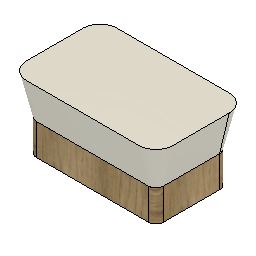
ZoomMuter_case_v13 (Autodesk Fusion 360 design; units mm, degrees)
Autodesk Fusion 360 part; units mm, degrees
note: some values were not read from the file. Set by a fixed rule: which sketch regions a step uses.
sketch "Sketch1" plane through (0, 0, 0) normal (0, 1, 0) x (1, 0, 0) in component "Case Front"
  line L0 (-27, 12.5) -> (-2, 12.5) construction
  line L1 (-2, 12.5) -> (-2, -12.5) construction
  line L2 (-2, -12.5) -> (-27, -12.5) construction
  line L3 (-27, -12.5) -> (-27, 12.5) construction
  line L4 (69.0491, 0) -> (-60.982, 0) construction
  line L5 (0, 36.3934) -> (0, -35.5501) construction
  line L6 (0, 18.5) -> (-33, 18.5)
  line L7 (-33, 18.5) -> (-33, 0)
  line L8 (-33, -18.5) -> (-33, 0)
  line L9 (0, -18.5) -> (-33, -18.5)
  line L10 (0, 18.5) -> (33, 18.5)
  line L11 (33, 18.5) -> (33, 0)
  line L12 (33, -18.5) -> (33, 0)
  line L13 (0, -18.5) -> (33, -18.5)
  line L14 (-14.5, 12.5) -> (-14.5, -12.5) construction
  line L15 (-7.2, -7.3) -> (-21.8, -7.3) construction
  line L16 (-21.8, -7.3) -> (-21.8, 7.3) construction
  line L17 (-21.8, 7.3) -> (-7.2, 7.3) construction
  line L18 (-7.2, 7.3) -> (-7.2, -7.3) construction
  line L19 (-7.2, -7.3) -> (-21.8, 7.3) construction
  line L20 (-21.8, -7.3) -> (-7.2, 7.3) construction
  line L21 (-22.1, 7.6) -> (-6.9, 7.6)
  line L22 (-6.9, 7.6) -> (-6.9, -7.6)
  line L23 (-6.9, -7.6) -> (-22.1, -7.6)
  line L24 (-22.1, -7.6) -> (-22.1, 7.6)
  line L25 (22.1, 7.6) -> (6.9, 7.6)
  line L26 (22.1, -7.6) -> (22.1, 7.6)
  line L27 (6.9, 7.6) -> (6.9, -7.6)
  line L28 (6.9, -7.6) -> (22.1, -7.6)
  line L29 (-22.7, 8.2) -> (-6.3, 8.2)
  line L30 (-6.3, 8.2) -> (-6.3, -8.2)
  line L31 (-6.3, -8.2) -> (-22.7, -8.2)
  line L32 (-22.7, -8.2) -> (-22.7, 8.2)
  line L33 (6.3, -8.2) -> (22.7, -8.2)
  line L34 (6.3, 8.2) -> (6.3, -8.2)
  line L35 (22.7, 8.2) -> (6.3, 8.2)
  line L36 (22.7, -8.2) -> (22.7, 8.2)
  point P0 (-14.5, 0)
  dimension "d1" = 25
  dimension "d2" = 25
  dimension "d5" = 6
  dimension "d6" = 6
  dimension "d7" = 6
  dimension "d11" = 14.6
  dimension "d12" = 14.6
  dimension "d14" = 2
  dimension "d39" = -0.9
  constraint horizontal L0
  constraint vertical L1
  constraint horizontal L2
  constraint vertical L3
  constraint perpendicular L1 L4
  constraint coincident origin L4
  constraint perpendicular L4 L5
  constraint coincident origin L5
  constraint coincident L5 L6.start
  constraint perpendicular L5 L6
  constraint coincident L4 L7.end
  constraint perpendicular L4 L7
  constraint symmetric L4 L6.start L9.start
  constraint symmetric L4 L6.end L8.start
  constraint symmetric L4 L7.end L8.end
  constraint symmetric L5 L6.start L10.start
  constraint symmetric L5 L6.end L10.end
  constraint symmetric L5 L7.end L11.end
  constraint symmetric L5 L8.start L12.start
  constraint symmetric L5 L9.start L13.start
  constraint midpoint L0 L14.start
  constraint midpoint L2 L14.end
  constraint perpendicular L15 L16
  constraint parallel L15 L17
  constraint parallel L16 L18
  constraint horizontal L15
  constraint coincident L19 P0
  constraint coincident L20 P0
  constraint midpoint L14 P0
  constraint symmetric L5 L21.start L25.start
  constraint symmetric L5 L21.end L25.end
  constraint symmetric L5 L22.end L27.end
  constraint symmetric L5 L23.end L26.start
  constraint symmetric L5 L29.start L35.start
  constraint symmetric L5 L29.end L34.start
  constraint symmetric L5 L30.end L33.start
  constraint symmetric L5 L31.end L33.end
  measures "d1" distance of L0.start L0.end
  measures "d2" distance of L0.start L2.end
  measures "d5" distance of L3 L7
  measures "d6" distance of L0 L6
  measures "d7" distance of L2 L9
  measures "d11" distance of L16.end L17.end
  measures "d12" distance of L15.end L16.end
  measures "d14" distance of L1 L5
extrude "Extrude1" add sketch "Sketch1" along normal blind 12 contours L6 L7 L8 L9 L10 L11 L12 L13 | L29 L30 L31 L32 | L33 L34 L35 L36 makes body 1 in component "Case Front"
extrude "Extrude5" cut sketch "Sketch1" along normal blind 10.5 contours L29 L30 L31 L32 | L33 L34 L35 L36 bodies 1 in component "Case Front"
fillet "Fillet1" radius 4 4 edges at (-33, 6, -18.5) (-33, 6, 18.5) (33, 6, -18.5) (33, 6, 18.5) on bodies 1 in component "Case Front"
sketch "Sketch2" plane through (0, 12, 0) normal (0, 1, 0) x (-1, 0, 0) in component "Case Front"
  line L0 (-22.1, 7.6) -> (-6.9, 7.6)
  line L1 (-6.9, 7.6) -> (-6.9, -7.6)
  line L2 (-6.9, -7.6) -> (-22.1, -7.6)
  line L3 (-22.1, -7.6) -> (-22.1, 7.6)
  line L4 (6.9, 7.6) -> (22.1, 7.6)
  line L5 (22.1, 7.6) -> (22.1, -7.6)
  line L6 (22.1, -7.6) -> (6.9, -7.6)
  line L7 (6.9, -7.6) -> (6.9, 7.6)
  line L8 (29, 18.5) -> (-29, 18.5)
  line L9 (-33, 14.5) -> (-33, -14.5)
  line L10 (-29, -18.5) -> (29, -18.5)
  line L11 (33, -14.5) -> (33, 14.5)
  arc A0 (-29, 18.5) -> (-33, 14.5) centre (-29, 14.5) ccw
  arc A1 (-33, -14.5) -> (-29, -18.5) centre (-29, -14.5) ccw
  arc A2 (29, -18.5) -> (33, -14.5) centre (29, -14.5) ccw
  arc A3 (33, 14.5) -> (29, 18.5) centre (29, 14.5) ccw
  line L12 (31, -13.325) -> (31, 13.325)
  line L13 (27.825, 16.5) -> (-27.825, 16.5)
  line L14 (-31, 13.325) -> (-31, -13.325)
  line L15 (-27.825, -16.5) -> (27.825, -16.5)
  arc A4 (27.825, -16.5) -> (31, -13.325) centre (27.825, -13.325) ccw
  arc A5 (-31, -13.325) -> (-27.825, -16.5) centre (-27.825, -13.325) ccw
  arc A6 (-27.825, 16.5) -> (-31, 13.325) centre (-27.825, 13.325) ccw
  arc A7 (31, 13.325) -> (27.825, 16.5) centre (27.825, 13.325) ccw
  line L16 (31.2, -13.325) -> (31.2, 13.325)
  arc A8 (31.2, 13.325) -> (27.825, 16.7) centre (27.825, 13.325) ccw
  line L17 (27.825, 16.7) -> (-27.825, 16.7)
  arc A9 (-27.825, 16.7) -> (-31.2, 13.325) centre (-27.825, 13.325) ccw
  line L18 (-31.2, 13.325) -> (-31.2, -13.325)
  arc A10 (-31.2, -13.325) -> (-27.825, -16.7) centre (-27.825, -13.325) ccw
  line L19 (-27.825, -16.7) -> (27.825, -16.7)
  arc A11 (27.825, -16.7) -> (31.2, -13.325) centre (27.825, -13.325) ccw
  dimension "d26" = 2
  dimension "d27" = 2
  dimension "d28" = 2
  dimension "d29" = 3.175
  dimension "d56" = 2
  dimension "d57" = 0.2
  constraint parallel L11 L12
  constraint parallel L8 L13
  constraint parallel L9 L14
  constraint tangent L12 A4
  constraint tangent L15 A4
  constraint tangent L14 A5
  constraint tangent L15 A5
  constraint equal A4 A5
  constraint tangent L14 A6
  constraint tangent L13 A6
  constraint equal A4 A6
  constraint tangent L13 A7
  constraint tangent L12 A7
  constraint equal A4 A7
  measures "d26" distance of L9 L14
  measures "d27" distance of L8 L13
  measures "d28" distance of L11 L12
  measures "d29" radius of A4
  measures "d56" distance of L10 L15
extrude "Extrude4" add sketch "Sketch2" along normal blind 4.2 contours L8 L9 L10 L11 A0 A1 A2 A3 bodies 1 in component "Case Front"
ref_plane "WorkPlane1" through (0, 12, 0) normal (0, 1, 0) x (0, 0, 1) in component "Switch Mockup"
sketch "Sketch1 (2)" plane through (0, 12, 0) normal (0, 1, 0) x (1, 0, 0) in component "Switch Mockup"
  line L0 (-6.9, -7.6) -> (-22.1, -7.6)
  line L1 (-22.1, -7.6) -> (-22.1, 7.6)
  line L2 (-6.9, 7.6) -> (-6.9, -7.6)
  line L3 (22.1, -7.6) -> (6.9, -7.6)
  line L4 (6.9, -7.6) -> (6.9, 7.6)
  line L5 (6.9, 7.6) -> (22.1, 7.6)
  line L6 (22.1, 7.6) -> (22.1, -7.6)
  line L7 (-6.9, -7.6) -> (-22.1, -7.6)
  line L8 (-22.1, -7.6) -> (-22.1, 7.6)
  line L9 (-22.1, 7.6) -> (-6.9, 7.6)
  line L10 (-6.9, 7.6) -> (-6.9, -7.6)
  line L11 (-31.2, 13.325) -> (-31.2, -13.325)
  arc A0 (-31.2, -13.325) -> (-27.825, -16.7) centre (-27.825, -13.325) ccw
  line L12 (-27.825, -16.7) -> (27.825, -16.7)
  arc A1 (27.825, -16.7) -> (31.2, -13.325) centre (27.825, -13.325) ccw
  line L13 (31.2, -13.325) -> (31.2, 13.325)
  arc A2 (31.2, 13.325) -> (27.825, 16.7) centre (27.825, 13.325) ccw
  line L14 (27.825, 16.7) -> (-27.825, 16.7)
  arc A3 (-27.825, 16.7) -> (-31.2, 13.325) centre (-27.825, 13.325) ccw
extrude "Extrude1'" add sketch "Sketch1 (2)" along normal blind 7.93 separate body contours L0 L1 L2 L7 L8 L9 L10 | L3 L4 L5 L6 makes body 2 at (-17.0333, 12, 2.5333) makes body 3 at (17.0333, 12, 2.5333) in component "Switch Mockup"
sketch "Sketch2 (2)" plane through (0, 19.93, 0) normal (0, 1, 0) x (-1, 0, 0) in component "Switch Mockup"
  line L0 (-22.1, -7.6) -> (-6.9, -7.6)
  line L1 (-6.9, -7.6) -> (-6.9, 7.6)
  line L2 (-6.9, 7.6) -> (-22.1, 7.6)
  line L3 (-22.1, 7.6) -> (-22.1, -7.6)
  circle A0 centre (15.2785, -5.9827) radius 1.0884
  circle A1 centre (15.2785, 4.052) radius 1.6496
  circle A2 centre (-14.7915, -5.9827) radius 0.7885
  circle A3 centre (-14.7915, 4.5657) radius 0.8169
extrude "Extrude2" add sketch "Sketch2 (2)" along normal blind 3.4 contours A0 | A1 | A2 | A3 bodies 2 3 in component "Switch Mockup"
ref_plane "WorkPlane1" through (0, 37, 0) normal (0, -1, 0) x (-1, 0, 0) in component "Case Back"
sketch "Sketch5" plane through (0, 16.2, 0) normal (0, 1, 0) x (-1, 0, 0) in component "Case Back"
  arc A0 (33, 14.5) -> (29, 18.5) centre (29, 14.5) ccw
  line L0 (29, 18.5) -> (-29, 18.5)
  arc A1 (-29, 18.5) -> (-33, 14.5) centre (-29, 14.5) ccw
  line L1 (-33, 14.5) -> (-33, -14.5)
  arc A2 (-33, -14.5) -> (-29, -18.5) centre (-29, -14.5) ccw
  line L2 (-29, -18.5) -> (29, -18.5)
  arc A3 (29, -18.5) -> (33, -14.5) centre (29, -14.5) ccw
  line L3 (33, -14.5) -> (33, 14.5)
  line L4 (-29, -18.5) -> (29, -18.5)
  arc A4 (29, -18.5) -> (33, -14.5) centre (29, -14.5) ccw
  line L5 (33, -14.5) -> (33, 14.5)
  arc A5 (33, 14.5) -> (29, 18.5) centre (29, 14.5) ccw
  line L6 (29, 18.5) -> (-29, 18.5)
  arc A6 (-29, 18.5) -> (-33, 14.5) centre (-29, 14.5) ccw
  line L7 (-33, 14.5) -> (-33, -14.5)
  arc A7 (-33, -14.5) -> (-29, -18.5) centre (-29, -14.5) ccw
sketch "Sketch4" plane through (0, 37, 0) normal (0, -1, 0) x (1, 0, 0) in component "Case Back"
  arc A0 (-29, 18.5) -> (-33, 14.5) centre (-29, 14.5) ccw
  line L0 (-29, 18.5) -> (29, 18.5)
  arc A1 (33, 14.5) -> (29, 18.5) centre (29, 14.5) ccw
  line L1 (33, 14.5) -> (33, -14.5)
  arc A2 (29, -18.5) -> (33, -14.5) centre (29, -14.5) ccw
  line L2 (29, -18.5) -> (-29, -18.5)
  arc A3 (-33, -14.5) -> (-29, -18.5) centre (-29, -14.5) ccw
  line L3 (-33, -14.5) -> (-33, 14.5)
  line L4 (29, -23.5) -> (-29, -23.5)
  arc A4 (-38, -14.5) -> (-29, -23.5) centre (-29, -14.5) ccw
  line L5 (-38, -14.5) -> (-38, 14.5)
  arc A5 (-29, 23.5) -> (-38, 14.5) centre (-29, 14.5) ccw
  line L6 (-29, 23.5) -> (29, 23.5)
  arc A6 (38, 14.5) -> (29, 23.5) centre (29, 14.5) ccw
  line L7 (38, 14.5) -> (38, -14.5)
  arc A7 (29, -23.5) -> (38, -14.5) centre (29, -14.5) ccw
  arc A8 (-29, 19.8) -> (-34.3, 14.5) centre (-29, 14.5) ccw
  line L8 (-34.3, -14.5) -> (-34.3, 14.5)
  arc A9 (-34.3, -14.5) -> (-29, -19.8) centre (-29, -14.5) ccw
  line L9 (29, -19.8) -> (-29, -19.8)
  arc A10 (29, -19.8) -> (34.3, -14.5) centre (29, -14.5) ccw
  line L10 (34.3, 14.5) -> (34.3, -14.5)
  arc A11 (34.3, 14.5) -> (29, 19.8) centre (29, 14.5) ccw
  line L11 (-29, 19.8) -> (29, 19.8)
  arc A12 (-31.2, -13.325) -> (-27.825, -16.7) centre (-27.825, -13.325) ccw
  line L12 (-27.825, -16.7) -> (27.825, -16.7)
  arc A13 (27.825, -16.7) -> (31.2, -13.325) centre (27.825, -13.325) ccw
  line L13 (31.2, -13.325) -> (31.2, 13.325)
  arc A14 (31.2, 13.325) -> (27.825, 16.7) centre (27.825, 13.325) ccw
  line L14 (27.825, 16.7) -> (-27.825, 16.7)
  arc A15 (-27.825, 16.7) -> (-31.2, 13.325) centre (-27.825, 13.325) ccw
  line L15 (-31.2, 13.325) -> (-31.2, -13.325)
  dimension "d33" = 5
  dimension "d35" = 1.3
loft "Loft1" add profiles "Sketch5", "Sketch4" section 1 section 2 contours L4 A4 L5 A5 L6 A6 L7 A7 separate body makes body 4 in component "Case Back"
shell "Shell2" thickness 3.7 removed faces 1 at (9.6667, 16.2, 6.1667) on bodies 4 in component "Case Back"
sketch "Sketch1 (3)" plane through (0, 16.2, 0) normal (0, 1, 0) x (-1, 0, 0) in component "Case Back"
  spline S0 degree 3 poles (-29.2013, -14.5) (-29.2013, -14.5015) (-29.2013, -14.506) (-29.2003, -14.5252) (-29.1983, -14.5383) (-29.1919, -14.5634) (-29.1875, -14.5752) (-29.1704, -14.6109) (-29.1539, -14.6321) (-29.1161, -14.6665) (-29.0934, -14.6807) (-29.0493, -14.6966) (-29.0305, -14.7) (-29.0089, -14.7011) (-29.0062, -14.7012) (-29.0025, -14.7013) (-29.0016, -14.7013) (-29.0005, -14.7013) (-29.0003, -14.7013) (-29, -14.7013) (-29, -14.7013) (-18.9136, -14.7013) (-9.2644, -14.7013) (5.7641, -14.7013) (11.2782, -14.7013) (19.004, -14.7013) (21.3301, -14.7013) (24.5877, -14.7013) (25.5676, -14.7013) (27.1216, -14.7013) (27.7083, -14.7013) (28.4749, -14.7013) (28.6696, -14.7013) (28.9056, -14.7013) (28.9526, -14.7013) (29.0022, -14.7013) (29.0085, -14.7012) (29.0298, -14.6997) (29.0426, -14.6974) (29.0674, -14.6905) (29.0791, -14.6859) (29.1146, -14.668) (29.1355, -14.6509) (29.1687, -14.6128) (29.1825, -14.5899) (29.1977, -14.5448) (29.2006, -14.5257) (29.2013, -14.5033) (29.2013, -14.5008) (29.2013, -9.4558) (29.2013, -4.6309) (29.2013, 2.8835) (29.2013, 5.6405) (29.2013, 9.5033) (29.2013, 10.6662) (29.2013, 12.4661) (29.2013, 13.1197) (29.2013, 14.0018) (29.2013, 14.2453) (29.2013, 14.4833) (29.2013, 14.4874) (29.2013, 14.5018) (29.2013, 14.5057) (29.2003, 14.5248) (29.1984, 14.5379) (29.192, 14.5631) (29.1877, 14.5748) (29.1707, 14.6105) (29.1542, 14.6318) (29.1164, 14.6663) (29.0937, 14.6805) (29.0497, 14.6965) (29.0309, 14.6999) (29.0094, 14.7011) (29.0066, 14.7012) (29.003, 14.7012) (29.002, 14.7013) (29.0005, 14.7013) (29, 14.7013) (13.9982, 14.7013) (-0.351, 14.7013) (-18.5064, 14.7013) (-22.6948, 14.7013) (-27.3011, 14.7013) (-27.8606, 14.7013) (-28.5398, 14.7013) (-28.6756, 14.7013) (-28.8435, 14.7013) (-28.8795, 14.7013) (-28.9316, 14.7013) (-28.9484, 14.7013) (-29.0028, 14.7013) (-29.005, 14.7013) (-29.0235, 14.7005) (-29.0366, 14.6986) (-29.0619, 14.6924) (-29.0737, 14.6881) (-29.1095, 14.6713) (-29.1308, 14.655) (-29.1656, 14.6174) (-29.1799, 14.5947) (-29.1962, 14.5509) (-29.1997, 14.5322) (-29.2013, 14.5066) (-29.2013, 14.4995) (-29.2013, 9.6328) (-29.2013, 4.8164) (-29.2013, 0) (-29.2013, -5.0431) (-29.2013, -9.8677) (-29.2013, -14.5) knots 1.51292242 1.51292242 1.51292242 1.51292242 1.51341061 1.51341061 1.51468048 1.51468048 1.51598415 1.51598415 1.51896361 1.51896361 1.52201263 1.52201263 1.52434216 1.52434216 1.52469932 1.52469932 1.52483423 1.52483423 1.52486538 1.52486538 1.52487073 1.52487073 1.86604744 1.86604744 2.07830234 2.07830234 2.17578069 2.17578069 2.2204858 2.2204858 2.2496217 2.2496217 2.26014609 2.26014609 2.26291297 2.26291297 2.26318968 2.26318968 2.26368981 2.26368981 2.26421181 2.26421181 2.26540782 2.26540782 2.26659472 2.26659472 2.26750254 2.26750254 2.26767067 2.26767067 2.77651558 2.77651558 3.09305783 3.09305783 3.23842388 3.23842388 3.32736932 3.32736932 3.36344051 3.36344051 3.36409413 3.36409413 3.36586679 3.36586679 3.37067589 3.37067589 3.37560507 3.37560507 3.38686687 3.38686687 3.39841677 3.39841677 3.4072384 3.4072384 3.40858843 3.40858843 3.409115 3.409115 3.40942694 3.40942694 5.06474265 5.06474265 5.59075846 5.59075846 5.66725479 5.66725479 5.68746684 5.68746684 5.69329523 5.69329523 5.69626231 5.69626231 5.70328303 5.70328303 5.72519357 5.72519357 5.74753972 5.74753972 5.79854212 5.79854212 5.8511881 5.8511881 5.89135844 5.89135844 5.90648228 5.90648228 7.35139546 7.35139546 7.35139546 8.86431788 8.86431788 8.86431788 8.86431788
  spline S1 degree 3 poles (-33, -14.5) (-33, -15.0365) (-32.8906, -15.5727) (-32.6806, -16.0663) (-32.5243, -16.4335) (-32.3127, -16.7771) (-32.0551, -17.0819) (-31.6766, -17.5299) (-31.1981, -17.893) (-30.6648, -18.1371) (-30.1444, -18.3753) (-29.5724, -18.5) (-29, -18.5) (-16.7583, -18.5) (16.7583, -18.5) (29, -18.5) (29.5365, -18.5) (30.0727, -18.3906) (30.5663, -18.1806) (30.9335, -18.0243) (31.2771, -17.8127) (31.5819, -17.5551) (32.0299, -17.1766) (32.393, -16.6981) (32.6371, -16.1648) (32.8753, -15.6444) (33, -15.0724) (33, -14.5) (33, -8.3792) (33, 8.3792) (33, 14.5) (33, 15.0365) (32.8906, 15.5727) (32.6806, 16.0663) (32.5243, 16.4335) (32.3127, 16.7771) (32.0551, 17.0819) (31.6766, 17.5299) (31.1981, 17.893) (30.6648, 18.1371) (30.1444, 18.3753) (29.5724, 18.5) (29, 18.5) (16.7583, 18.5) (-16.7583, 18.5) (-29, 18.5) (-29.5365, 18.5) (-30.0727, 18.3906) (-30.5663, 18.1806) (-30.9335, 18.0243) (-31.2771, 17.8127) (-31.5819, 17.5551) (-32.0299, 17.1766) (-32.393, 16.6981) (-32.6371, 16.1648) (-32.8753, 15.6444) (-33, 15.0724) (-33, 14.5) (-33, 8.3792) (-33, -8.3792) (-33, -14.5) knots 0 0 0 0 0.011894 0.011894 0.011894 0.020742 0.020742 0.020742 0.033746 0.033746 0.033746 0.046436 0.046436 0.046436 0.317855 0.317855 0.317855 0.329749 0.329749 0.329749 0.338597 0.338597 0.338597 0.351601 0.351601 0.351601 0.364291 0.364291 0.364291 0.5 0.5 0.5 0.511894 0.511894 0.511894 0.520742 0.520742 0.520742 0.533746 0.533746 0.533746 0.546436 0.546436 0.546436 0.817855 0.817855 0.817855 0.829749 0.829749 0.829749 0.838597 0.838597 0.838597 0.851601 0.851601 0.851601 0.864291 0.864291 0.864291 1 1 1 1
  arc A0 (27.825, -16.5) -> (31, -13.325) centre (27.825, -13.325) ccw
  line L0 (-27.825, -16.5) -> (27.825, -16.5)
  line L1 (31, -13.325) -> (31, 13.325)
  arc A1 (31, 13.325) -> (27.825, 16.5) centre (27.825, 13.325) ccw
  line L2 (27.825, 16.5) -> (-27.825, 16.5)
  arc A2 (-27.825, 16.5) -> (-31, 13.325) centre (-27.825, 13.325) ccw
  line L3 (-31, 13.325) -> (-31, -13.325)
  arc A3 (-31, -13.325) -> (-27.825, -16.5) centre (-27.825, -13.325) ccw
  line L4 (30.8, -13.325) -> (30.8, 13.325)
  arc A4 (30.8, 13.325) -> (27.825, 16.3) centre (27.825, 13.325) ccw
  line L5 (27.825, 16.3) -> (-27.825, 16.3)
  arc A5 (-27.825, 16.3) -> (-30.8, 13.325) centre (-27.825, 13.325) ccw
  line L6 (-30.8, 13.325) -> (-30.8, -13.325)
  arc A6 (-30.8, -13.325) -> (-27.825, -16.3) centre (-27.825, -13.325) ccw
  line L7 (-27.825, -16.3) -> (27.825, -16.3)
  arc A7 (27.825, -16.3) -> (30.8, -13.325) centre (27.825, -13.325) ccw
  arc A8 (27.825, -16.7) -> (31.2, -13.325) centre (27.825, -13.325) ccw
  line L8 (27.825, -16.7) -> (-27.825, -16.7)
  arc A9 (-31.2, -13.325) -> (-27.825, -16.7) centre (-27.825, -13.325) ccw
  line L9 (-31.2, -13.325) -> (-31.2, 13.325)
  arc A10 (-27.825, 16.7) -> (-31.2, 13.325) centre (-27.825, 13.325) ccw
  line L10 (-27.825, 16.7) -> (27.825, 16.7)
  arc A11 (31.2, 13.325) -> (27.825, 16.7) centre (27.825, 13.325) ccw
  line L11 (31.2, 13.325) -> (31.2, -13.325)
  arc A12 (33, 14.5) -> (29, 18.5) centre (29, 14.5) ccw
  line L12 (29, 18.5) -> (-29, 18.5)
  arc A13 (-29, 18.5) -> (-33, 14.5) centre (-29, 14.5) ccw
  line L13 (-33, 14.5) -> (-33, -14.5)
  arc A14 (-33, -14.5) -> (-29, -18.5) centre (-29, -14.5) ccw
  line L14 (-29, -18.5) -> (29, -18.5)
  arc A15 (29, -18.5) -> (33, -14.5) centre (29, -14.5) ccw
  line L15 (33, -14.5) -> (33, 14.5)
extrude "Extrude4'" add sketch "Sketch1 (3)" against normal up to surface (4.2 mm away) separate body contours L4 A4 L5 A5 L6 A6 L7 A7 makes body 5 in component "Case Back"
component "Case Front" placed x (1, 0, 0) y (0, 1, 0) z (0, 0, 1) at (0, 0, 0)
component "Switch Mockup" placed x (1, 0, 0) y (0, 1, 0) z (0, 0, 1) at (0, 0, 0)
component "Case Back" placed x (1, 0, 0) y (0, 1, 0) z (0, 0, 1) at (0, 0, 0)
equation "key_sidel = 14.6 mm"
equation "key_tolerance = 0.3 mm"
equation "d11 = key_sidel"
equation "d12 = key_sidel"
equation "d13 = -key_tolerance"
equation "d14 = ( 4 / 2 ) * 1 mm"
equation "d15 = front_height + catch_height"
equation "d29 = 1 / 8 * 1 in"
equation "d30 = 1 / 2 * 1 in - 9.2 mm + 0.7 mm"
equation "d35 = 5 mm - 3.7 mm"
equation "d39 = -key_tolerance - 0.6 mm"
equation "d40 = front_height"
equation "fit_tolerance_bottom = 0.2 mm"
equation "catch_height = 1.5 mm"
equation "fit_tolerance_top = 0.2 mm"
equation "d57 = fit_tolerance_top"
equation "d60 = -fit_tolerance_bottom"
equation "front_height = 10.7 mm - 2.5 mm + 2.3 mm"
